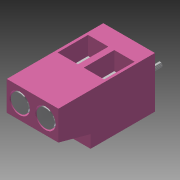
# Autodesk Inventor part: ScrewTerminal
Saved by Autodesk Inventor 2014 (Build 180170000, 170)
## iProperties
Created: 2015-04-18
Part Number: ScrewTerminal
Material: Generic
Document SubType Name: Modeling
Designer: Owner
Density: 1 g/cm^3
Appearance: Pink
Author: Owner
Autodesk Inventor part; units mm, degrees
ref_plane "YZ Plane" through (0, 0, 0) normal (1, 0, 0) x (0, 1, 0)
ref_plane "XZ Plane" through (0, 0, 0) normal (0, 1, 0) x (-1, 0, 0)
ref_plane "XY Plane" through (0, 0, 0) normal (0, 0, 1) x (1, 0, 0)
sketch "Sketch1" plane through (0, 0, 0) normal (1, 0, 0) x (0, 1, 0)
  line L0 (-6.9022, 3.3081) -> (3.0978, 3.3081)
  line L1 (3.0978, 3.3081) -> (3.0978, -9.3586)
  line L2 (3.0978, -9.3586) -> (-6.9022, -9.3586)
  line L3 (-6.9022, -9.3586) -> (-6.9022, 3.3081)
  line L4 (-4.3921, 3.3081) -> (-2.6747, 9.6414)
  line L5 (-2.6747, 9.6414) -> (3.0978, 9.6414)
  line L6 (3.0978, 9.6414) -> (3.0978, 3.3081)
  point P0 (0, 0)
  dimension "d0" = 10
  dimension "d1" = 19
  dimension "d2" = 12.6667
  constraints: 14 end point, 3 perpendicular, 2 parallel, 1 horizontal, 1 point on line
  measures "d0" distance between parallel lines of L1 L3
  measures "d1" distance between parallel lines of L2 L5
  measures "d2" distance between parallel lines of L2 L0
extrude "Extrusion1" add sketch "Sketch1" along normal blind 10.16
sketch "Sketch2" plane through (0, -6.9022, -9.3586) normal (0, 0, -1) x (-1, 0, 0)
  line L0 (-10.16, 0) -> (-10.16, 10) projected
  line L1 (0, 0) -> (-10.16, 0) projected
  circle A0 centre (-7.62, 5) radius 0.45
  circle A1 centre (-2.54, 5) radius 0.45
  point P0 (0, 6.9022)
  dimension "d5" = 0.9
  dimension "d6" = 0.9
  dimension "d7" = 5.08
  dimension "d8" = 2.54
  dimension "d9" = 5
  dimension "d10" = 5
  constraints: 2 centre point
  measures "d5" diameter of A0
  measures "d6" diameter of A1
  measures "d7" distance of A1.centre A0.centre
  measures "d8" distance from line of L0 A0.centre
  measures "d9" distance from line of L1 A0.centre
  measures "d10" distance from line of L1 A1.centre
extrude "Extrusion2" add sketch "Sketch2" along normal blind 3.6
sketch "Sketch3" plane through (0, -2.6747, 9.6414) normal (0, 0, 1) x (1, 0, 0)
  line L0 (0, 5.7725) -> (0, 0) projected
  circle A0 centre (2.54, 2.8863) radius 2
  circle A1 centre (7.62, 2.8863) radius 2
  point P0 (0, 2.6747)
  dimension "d13" = 5.08
  dimension "d14" = 4
  dimension "d15" = 4
  dimension "d16" = 2.54
  constraints: 2 centre point
  measures "d13" distance of A1.centre A0.centre
  measures "d14" diameter of A1
  measures "d15" diameter of A0
  measures "d16" distance from line of L0 A0.centre
extrude "Extrusion3" cut sketch "Sketch3" against normal blind 3.6
sketch "Sketch4" plane through (2.54, 0.2116, 6.0414) normal (0, 0, 1) x (1, 0, 0)
  circle A0 centre (0, 0) radius 2 projected
  circle A1 centre (0, 0) radius 1.75
  circle A2 centre (5.08, 0) radius 1.75
  point P0 (-2.54, -0.2116)
  dimension "d19" = 5.08
  dimension "d20" = 3.5
  dimension "d21" = 3.5
  constraints: 2 centre point, 1 coincident
  measures "d19" distance of A2.centre A1.centre
  measures "d20" diameter of A1
  measures "d21" diameter of A2
extrude "Extrusion4" add sketch "Sketch4" along normal blind 3.6 contours A1 | A2
sketch "Sketch5" plane through (0, 3.0978, 9.6414) normal (0, 1, 0) x (1, 0, 0)
  line L0 (0, 19) -> (0, 0) projected
  line L1 (10.16, 19) -> (10.16, 0) projected
  line L2 (0, 19) -> (10.16, 19) projected
  line L3 (0.5, 15.5) -> (4.5, 15.5)
  line L4 (4.5, 15.5) -> (4.5, 9.5)
  line L5 (4.5, 9.5) -> (0.5, 9.5)
  line L6 (0.5, 9.5) -> (0.5, 15.5)
  line L7 (5.66, 15.5) -> (9.66, 15.5)
  line L8 (9.66, 15.5) -> (9.66, 9.5)
  line L9 (9.66, 9.5) -> (5.66, 9.5)
  line L10 (5.66, 9.5) -> (5.66, 15.5)
  point P0 (0, 9.6414)
  dimension "d24" = 4
  dimension "d25" = 4
  dimension "d26" = 0.5
  dimension "d27" = 0.5
  dimension "d28" = 3.5
  dimension "d29" = 3.5
  dimension "d30" = 6
  dimension "d31" = 6
  constraints: 16 end point, 4 parallel, 2 horizontal, 2 perpendicular
  measures "d24" distance of L3.start L3.end
  measures "d25" distance of L7.start L7.end
  measures "d26" distance between parallel lines of L0 L6
  measures "d27" distance between parallel lines of L1 L8
  measures "d28" distance between parallel lines of L2 L3
  measures "d29" distance between parallel lines of L7 L2
  measures "d30" distance of L5.end L3.start
  measures "d31" distance of L7.end L8.end
extrude "Extrusion5" cut sketch "Sketch5" against normal blind 3.6
body "Solid1"
